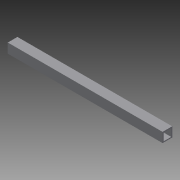
# Autodesk Inventor part: alignmentWheelsBarSolid
Saved by Autodesk Inventor 2015 (Build 190159000, 159)
## iProperties
Created: 2015-01-30
Part Number: alignmentWheelsBarSolid
Material: Generic
Document SubType Name: Modeling
Designer: Kingbob26
Density: 1 g/cm^3
Appearance: Default
Author: Kingbob26
Autodesk Inventor part; units mm, degrees
ref_plane "YZ Plane" through (0, 0, 0) normal (1, 0, 0) x (0, 1, 0)
ref_plane "XZ Plane" through (0, 0, 0) normal (0, 1, 0) x (-1, 0, 0)
ref_plane "XY Plane" through (0, 0, 0) normal (0, 0, 1) x (1, 0, 0)
sketch "Sketch1" plane through (0, 0, 0) normal (0, 1, 0) x (-1, 0, 0)
  line L0 (381, 15.875) -> (-381, 15.875)
  line L1 (-381, 15.875) -> (-381, -15.875)
  line L2 (-381, -15.875) -> (381, -15.875)
  line L3 (381, -15.875) -> (381, 15.875)
  point P0 (0, 0)
  dimension "d0" = 762
  dimension "d1" = 31.75
  constraints: 8 end point, 2 parallel, 1 horizontal, 1 perpendicular
  measures "d0" distance of L2.end L1.end
  measures "d1" distance of L1.end L0.end
extrude "Extrusion1" add sketch "Sketch1" along normal blind 3.175
sketch "Sketch2" plane through (-381, 0, 15.875) normal (0, 0, 1) x (1, 0, 0)
  line L0 (0, 3.175) -> (762, 3.175) projected
  line L1 (762, 28.575) -> (0, 28.575)
  line L2 (0, 28.575) -> (0, 3.175)
  line L3 (0, 3.175) -> (762, 3.175)
  line L4 (762, 3.175) -> (762, 28.575)
  point P0 (381, 0)
  constraints: 8 end point, 2 parallel, 1 horizontal, 1 perpendicular
extrude "Extrusion2" add sketch "Sketch2" against normal blind 3.175
sketch "Sketch3" plane through (-381, 28.575, 15.875) normal (0, 1, 0) x (1, 0, 0)
  line L0 (0, 3.175) -> (762, 3.175) projected
  line L1 (762, 28.575) -> (0, 28.575)
  line L2 (0, 28.575) -> (0, 3.175)
  line L3 (0, 3.175) -> (762, 3.175)
  line L4 (762, 3.175) -> (762, 28.575)
  point P0 (381, 15.875)
  constraints: 8 end point, 2 parallel, 1 horizontal, 1 perpendicular
extrude "Extrusion3" add sketch "Sketch3" against normal blind 3.175
sketch "Sketch4" plane through (381, 28.575, -12.7) normal (0, 0, -1) x (-1, 0, 0)
  line L0 (762, 0) -> (0, 0) projected
  line L1 (0, -25.4) -> (762, -25.4) projected
  line L2 (0, -3.175) -> (0, -25.4) projected
  line L3 (762, -25.4) -> (762, -3.175) projected
  line L4 (762, 0) -> (0, 0)
  line L5 (0, 0) -> (0, -25.4)
  line L6 (0, -25.4) -> (762, -25.4)
  line L7 (762, -25.4) -> (762, 0)
  point P0 (381, -28.575)
  constraints: 8 end point, 2 parallel, 1 horizontal, 1 perpendicular
extrude "Extrusion4" add sketch "Sketch4" along normal blind 3.175
sketch "Sketch5" plane through (-381, 28.575, 15.875) normal (0, 1, 0) x (1, 0, 0)
  line L0 (0, 31.75) -> (762, 31.75) projected
  line L1 (0, 0) -> (762, 0) projected
  line L2 (762, 0) -> (762, 31.75) projected
  line L3 (0, 31.75) -> (762, 31.75) projected
  line L4 (0, 0) -> (0, 31.75) projected
  line L5 (0, 31.75) -> (762, 31.75)
  line L6 (762, 31.75) -> (762, 0)
  line L7 (762, 0) -> (0, 0)
  line L8 (0, 0) -> (0, 31.75)
  point P0 (381, 15.875)
  constraints: 8 end point, 2 parallel, 1 horizontal, 1 perpendicular
extrude "Extrusion5" add sketch "Sketch5" along normal blind 3.175
sketch "Sketch6" plane through (-381, 25.4, 15.875) normal (0, -1, 0) x (1, 0, 0)
  line L0 (0, -3.175) -> (0, -28.575) projected
  line L1 (0, -28.575) -> (762, -28.575) projected
  line L2 (762, -28.575) -> (762, -3.175) projected
  line L3 (0, -3.175) -> (762, -3.175) projected
  line L4 (762, -3.175) -> (0, -3.175)
  line L5 (0, -3.175) -> (0, -28.575)
  line L6 (0, -28.575) -> (762, -28.575)
  line L7 (762, -28.575) -> (762, -3.175)
  point P0 (381, -15.875)
  constraints: 8 end point, 2 parallel, 1 horizontal, 1 perpendicular
extrude "Extrusion6" cut sketch "Sketch6" against normal blind 3.175
sketch "Sketch7" plane through (381, 0, 15.875) normal (1, 0, 0) x (0, 0, -1)
  line L0 (0, 31.75) -> (31.75, 31.75) projected
  line L1 (31.75, 0) -> (31.75, 31.75) projected
  line L2 (0, 31.75) -> (31.75, 31.75) projected
  line L3 (0, 0) -> (0, 31.75) projected
  line L4 (0, 0) -> (31.75, 0) projected
  line L5 (3.175, 28.575) -> (3.175, 3.175) projected
  line L6 (3.175, 28.575) -> (28.575, 28.575) projected
  line L7 (28.575, 28.575) -> (28.575, 3.175) projected
  line L8 (3.175, 3.175) -> (28.575, 3.175) projected
  line L9 (0, 0) -> (0, 31.75) projected
  line L10 (0, 31.75) -> (31.75, 31.75)
  line L11 (31.75, 31.75) -> (31.75, 0)
  line L12 (31.75, 0) -> (0, 0)
  line L13 (0, 0) -> (0, 31.75)
  line L14 (3.175, 28.575) -> (28.575, 28.575)
  line L15 (28.575, 28.575) -> (28.575, 3.175)
  line L16 (28.575, 3.175) -> (3.175, 3.175)
  line L17 (3.175, 3.175) -> (3.175, 28.575)
  point P0 (15.875, 0)
  constraints: 16 end point, 4 parallel, 2 horizontal, 2 perpendicular
extrude "Extrusion7" cut sketch "Sketch7" against normal blind 254
body "Solid1"
